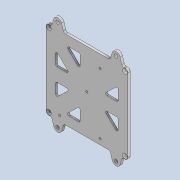
# Autodesk Inventor part: sacatola coperchio principale
Saved by Autodesk Inventor 2022 (Build 260153000, 153)
## iProperties
Created: 2025-07-12
Part Number: sacatola coperchio principale
Material: Generic
Document SubType Name: Modeling
Designer: 1234
Density: 1 g/cm^3
Appearance: Default
Author: 1234
Autodesk Inventor part; units mm, degrees
ref_plane "YZ Plane" through (0, 0, 0) normal (1, 0, 0) x (0, 1, 0)
ref_plane "XZ Plane" through (0, 0, 0) normal (0, 1, 0) x (-1, 0, 0)
ref_plane "XY Plane" through (0, 0, 0) normal (0, 0, 1) x (1, 0, 0)
sketch "Sketch1" plane through (0, 0, 0) normal (0, 0, 1) x (1, 0, 0)
  arc A0 (116, 108) -> (112, 112) centre (112, 108) ccw
  circle A1 centre (112, 108) radius 4 construction
  arc A2 (112, -4) -> (116, 0) centre (112, 0) ccw
  circle A3 centre (112, 0) radius 4 construction
  arc A4 (-4, 0) -> (0, -4) centre (0, 0) ccw
  circle A5 centre (0, 0) radius 4 construction
  arc A6 (0, 112) -> (-4, 108) centre (0, 108) ccw
  circle A7 centre (0, 108) radius 4 construction
  line L0 (0, 108) -> (112, 108) construction
  line L1 (112, 108) -> (112, 0) construction
  line L2 (112, 0) -> (0, 0) construction
  line L3 (0, 0) -> (0, 108) construction
  circle A8 centre (112, 0) radius 1.6
  circle A9 centre (0, 0) radius 1.6
  circle A10 centre (0, 108) radius 1.6
  circle A11 centre (112, 108) radius 1.6
  line L4 (116, 108) -> (116, 0)
  line L5 (112, 112) -> (0, 112)
  line L6 (-4, 108) -> (-4, 0)
  line L7 (0, -4) -> (112, -4)
  line L8 (6, -2) -> (106, -2)
  line L9 (106, -2) -> (6, -2)
  line L10 (-2, 6) -> (-2, 102)
  line L11 (-2, 6) -> (-2, 102)
  line L12 (106, 110) -> (6, 110)
  line L13 (6, 110) -> (106, 110)
  line L14 (114, 6) -> (114, 102)
  line L15 (114, 102) -> (114, 6)
  arc A12 (6, 110) -> (4, 108) centre (6, 108) ccw
  arc A13 (6, 110) -> (4, 108) centre (6, 108) ccw
  arc A14 (0, 104) -> (-2, 102) centre (0, 102) ccw
  arc A15 (0, 104) -> (4, 108) centre (0, 108) ccw
  arc A16 (0, 104) -> (4, 108) centre (0, 108) ccw
  arc A17 (0, 104) -> (-2, 102) centre (0, 102) ccw
  arc A18 (114, 102) -> (112, 104) centre (112, 102) ccw
  arc A19 (114, 102) -> (112, 104) centre (112, 102) ccw
  arc A20 (108, 108) -> (112, 104) centre (112, 108) ccw
  arc A21 (108, 108) -> (112, 104) centre (112, 108) ccw
  arc A22 (108, 108) -> (106, 110) centre (106, 108) ccw
  arc A23 (108, 108) -> (106, 110) centre (106, 108) ccw
  arc A24 (112, 4) -> (114, 6) centre (112, 6) ccw
  arc A25 (112, 4) -> (114, 6) centre (112, 6) ccw
  arc A26 (112, 4) -> (108, 0) centre (112, 0) ccw
  arc A27 (112, 4) -> (108, 0) centre (112, 0) ccw
  arc A28 (106, -2) -> (108, 0) centre (106, 0) ccw
  arc A29 (106, -2) -> (108, 0) centre (106, 0) ccw
  arc A30 (4, 0) -> (6, -2) centre (6, 0) ccw
  arc A31 (4, 0) -> (6, -2) centre (6, 0) ccw
  arc A32 (-2, 6) -> (0, 4) centre (0, 6) ccw
  arc A33 (-2, 6) -> (0, 4) centre (0, 6) ccw
  arc A34 (4, 0) -> (0, 4) centre (0, 0) ccw
  arc A35 (4, 0) -> (0, 4) centre (0, 0) ccw
  arc A36 (-0.5, 6) -> (0, 5.5) centre (0, 6) ccw
  line L16 (-0.5, 6) -> (-0.5, 102)
  arc A37 (0, 102.5) -> (-0.5, 102) centre (0, 102) ccw
  arc A38 (0, 102.5) -> (5.5, 108) centre (0, 108) ccw
  arc A39 (6, 108.5) -> (5.5, 108) centre (6, 108) ccw
  line L17 (6, 108.5) -> (106, 108.5)
  arc A40 (106.5, 108) -> (106, 108.5) centre (106, 108) ccw
  arc A41 (106.5, 108) -> (112, 102.5) centre (112, 108) ccw
  arc A42 (112.5, 102) -> (112, 102.5) centre (112, 102) ccw
  line L18 (112.5, 102) -> (112.5, 6)
  arc A43 (112, 5.5) -> (112.5, 6) centre (112, 6) ccw
  arc A44 (112, 5.5) -> (106.5, 0) centre (112, 0) ccw
  arc A45 (106, -0.5) -> (106.5, 0) centre (106, 0) ccw
  line L19 (106, -0.5) -> (6, -0.5)
  arc A46 (5.5, 0) -> (6, -0.5) centre (6, 0) ccw
  arc A47 (5.5, 0) -> (0, 5.5) centre (0, 0) ccw
  arc A48 (-1, 6) -> (0, 5) centre (0, 6) ccw
  line L20 (-1, 6) -> (-1, 102)
  arc A49 (0, 103) -> (-1, 102) centre (0, 102) ccw
  arc A50 (0, 103) -> (5, 108) centre (0, 108) ccw
  arc A51 (6, 109) -> (5, 108) centre (6, 108) ccw
  line L21 (6, 109) -> (106, 109)
  arc A52 (107, 108) -> (106, 109) centre (106, 108) ccw
  arc A53 (107, 108) -> (112, 103) centre (112, 108) ccw
  arc A54 (113, 102) -> (112, 103) centre (112, 102) ccw
  line L22 (113, 102) -> (113, 6)
  arc A55 (112, 5) -> (113, 6) centre (112, 6) ccw
  arc A56 (112, 5) -> (107, 0) centre (112, 0) ccw
  arc A57 (106, -1) -> (107, 0) centre (106, 0) ccw
  line L23 (106, -1) -> (6, -1)
  arc A58 (5, 0) -> (6, -1) centre (6, 0) ccw
  arc A59 (5, 0) -> (0, 5) centre (0, 0) ccw
  arc A60 (-2.5, 6) -> (0, 3.5) centre (0, 6) ccw
  line L24 (-2.5, 6) -> (-2.5, 102)
  arc A61 (0, 104.5) -> (-2.5, 102) centre (0, 102) ccw
  arc A62 (0, 104.5) -> (3.5, 108) centre (0, 108) ccw
  arc A63 (6, 110.5) -> (3.5, 108) centre (6, 108) ccw
  line L25 (6, 110.5) -> (106, 110.5)
  arc A64 (108.5, 108) -> (106, 110.5) centre (106, 108) ccw
  arc A65 (108.5, 108) -> (112, 104.5) centre (112, 108) ccw
  arc A66 (114.5, 102) -> (112, 104.5) centre (112, 102) ccw
  line L26 (114.5, 102) -> (114.5, 6)
  arc A67 (112, 3.5) -> (114.5, 6) centre (112, 6) ccw
  arc A68 (112, 3.5) -> (108.5, 0) centre (112, 0) ccw
  arc A69 (106, -2.5) -> (108.5, 0) centre (106, 0) ccw
  line L27 (106, -2.5) -> (6, -2.5)
  arc A70 (3.5, 0) -> (6, -2.5) centre (6, 0) ccw
  arc A71 (3.5, 0) -> (0, 3.5) centre (0, 0) ccw
  line L28 (111.5, 6.4807) -> (111.5, 101.5193)
  arc A72 (105.5193, 107.5) -> (111.5, 101.5193) centre (112, 108) ccw
  line L29 (105.5193, 107.5) -> (6.4807, 107.5)
  arc A73 (0.5, 101.5193) -> (6.4807, 107.5) centre (0, 108) ccw
  line L30 (0.5, 101.5193) -> (0.5, 6.4807)
  arc A74 (6.4807, 0.5) -> (0.5, 6.4807) centre (0, 0) ccw
  line L31 (6.4807, 0.5) -> (105.5193, 0.5)
  arc A75 (111.5, 6.4807) -> (105.5193, 0.5) centre (112, 0) ccw
  line L32 (111.5, 6.4807) -> (111.5, 101.5193)
  arc A76 (105.5193, 107.5) -> (111.5, 101.5193) centre (112, 108) ccw
  line L33 (105.5193, 107.5) -> (6.4807, 107.5)
  arc A77 (0.5, 101.5193) -> (6.4807, 107.5) centre (0, 108) ccw
  line L34 (0.5, 101.5193) -> (0.5, 6.4807)
  arc A78 (6.4807, 0.5) -> (0.5, 6.4807) centre (0, 0) ccw
  line L35 (6.4807, 0.5) -> (105.5193, 0.5)
  arc A79 (111.5, 6.4807) -> (105.5193, 0.5) centre (112, 0) ccw
  line L36 (-0.5, 8) -> (1.5, 8)
  line L37 (1.5, 8) -> (1.5, 13)
  line L38 (1.5, 13) -> (-0.5, 13)
  line L39 (7, -0.5) -> (7, 1.5)
  line L40 (7, 1.5) -> (12, 1.5)
  line L41 (12, 1.5) -> (12, -0.5)
  line L42 (-4, 54) -> (-11, 54) construction
  circle A80 centre (-11, 54) radius 1.7
  arc A81 (-11, 58) -> (-11, 50) centre (-11, 54) ccw
  line L43 (-11, 50) -> (-4, 50)
  line L44 (-11, 58) -> (-4, 58)
  line L45 (7, -4) -> (7, -13) construction
  arc A82 (7, -13) -> (19, -13) centre (13, -13) ccw
  line L46 (19, -13) -> (19, -4)
  circle A83 centre (13, -13) radius 2.6
  line L47 (22, -4) -> (18.7417, -14.7417)
  line L48 (7, -13) -> (7, -4)
  line L49 (4, -4) -> (7.2583, -14.7417)
  line L50 (-12.4444, 50.2699) -> (-4, 47)
  line L51 (-12.4444, 57.7301) -> (-4, 61)
  line L52 (7, 112) -> (7, 121) construction
  arc A84 (19, 121) -> (7, 121) centre (13, 121) ccw
  line L53 (19, 121) -> (19, 112)
  circle A85 centre (13, 121) radius 2.6
  line L54 (22, 112) -> (18.7417, 122.7417)
  line L55 (7, 121) -> (7, 112)
  line L56 (4, 112) -> (7.2583, 122.7417)
  line L57 (99, -0.5) -> (99, 1.5)
  line L58 (99, 1.5) -> (104, 1.5)
  line L59 (104, 1.5) -> (104, -0.5)
  line L60 (56, -4) -> (56, -8.0114) construction
  line L61 (116, 54) -> (127.5654, 54) construction
  line L62 (53.5, -0.5) -> (53.5, 1.5)
  line L63 (53.5, 1.5) -> (58.5, 1.5)
  line L64 (58.5, 1.5) -> (58.5, -0.5)
  line L65 (112.5, 8) -> (110.5, 8)
  line L66 (110.5, 8) -> (110.5, 13)
  line L67 (110.5, 13) -> (112.5, 13)
  line L68 (-0.5, 100) -> (1.5, 100)
  line L69 (1.5, 100) -> (1.5, 95)
  line L70 (1.5, 95) -> (-0.5, 95)
  line L71 (7, 108.5) -> (7, 106.5)
  line L72 (7, 106.5) -> (12, 106.5)
  line L73 (12, 106.5) -> (12, 108.5)
  line L74 (99, 108.5) -> (99, 106.5)
  line L75 (99, 106.5) -> (104, 106.5)
  line L76 (104, 106.5) -> (104, 108.5)
  line L77 (53.5, 108.5) -> (53.5, 106.5)
  line L78 (53.5, 106.5) -> (58.5, 106.5)
  line L79 (58.5, 106.5) -> (58.5, 108.5)
  line L80 (112.5, 100) -> (110.5, 100)
  line L81 (110.5, 100) -> (110.5, 95)
  line L82 (110.5, 95) -> (112.5, 95)
  line L83 (13, -13) -> (13, -6.0057) construction
  point P0 (0, 0)
  point P1 (0.5, 13)
  point P2 (0.5, 8)
  point P3 (12, 0.5)
  point P4 (7, 0.5)
  point P5 (0.5, 13)
  point P6 (0.5, 8)
  point P7 (12, 0.5)
  point P8 (7, 0.5)
  point P9 (4, 112)
  point P10 (22, 104)
  point P11 (111.5, 100)
  point P12 (104, 107.5)
  point P13 (104, 100.5)
  point P14 (0.5, 95)
  point P15 (0.5, 95)
  point P16 (0.5, 100)
  point P17 (0.5, 100)
  point P18 (7, 107.5)
  point P19 (7, 107.5)
  point P20 (12, 107.5)
  point P21 (12, 107.5)
  point P22 (53.5, 107.5)
  point P23 (53.5, 107.5)
  point P24 (58.5, 107.5)
  point P25 (58.5, 107.5)
  point P26 (99, 107.5)
  point P27 (99, 107.5)
  point P28 (104, 107.5)
  point P29 (111.5, 100)
  point P30 (111.5, 95)
  point P31 (111.5, 95)
  point P32 (111.5, 13)
  point P33 (111.5, 13)
  point P34 (111.5, 8)
  point P35 (111.5, 8)
  point P36 (104, 0.5)
  point P37 (104, 0.5)
  point P38 (99, 0.5)
  point P39 (99, 0.5)
  point P40 (58.5, 0.5)
  point P41 (58.5, 0.5)
  point P42 (53.5, 0.5)
  point P43 (53.5, 0.5)
  point P44 (99, 130.5)
  point P45 (104, 130.5)
  point P46 (99, 120.5)
  point P47 (104, 120.5)
  dimension "d15" = 8
  dimension "d16" = 8
  dimension "d18" = 8
  dimension "d19" = 8
  dimension "d0" = 3.2
  dimension "d1" = 3.2
  dimension "d2" = 3.2
  dimension "d3" = 3.2
  dimension "d9" = 1.5
  dimension "d10" = 0.5
  dimension "d11" = 1.5
  dimension "d12" = 108
  dimension "d20" = 3.5
  dimension "d22" = 2.5
  dimension "d23" = 3.5
  dimension "d24" = 2.5
  dimension "d25" = 2.5
  dimension "d26" = 3.5
  dimension "d27" = 2.5
  dimension "d28" = 3.5
  dimension "d29" = 2.5
  dimension "d30" = 2.5
  dimension "d40" = 1
  dimension "d45" = 1
  dimension "d48" = 8
  dimension "d49" = 5
  dimension "d50" = 5
  dimension "d64" = 7
  dimension "d65" = 3.4
  dimension "d66" = 8
  dimension "d67" = 12
  dimension "d68" = 9
  dimension "d69" = 5.2
  dimension "d74" = 3
  dimension "d81" = 3
  dimension "d82" = 3
  dimension "d83" = 3
  dimension "d95" = 2
  dimension "d96" = 2
  dimension "d100" = 2
  dimension "d101" = 5
  dimension "d102" = 8
  dimension "d106" = 4.0114
  dimension "d107" = 11.5654
  dimension "d108" = 2
  dimension "d109" = 5
  dimension "d110" = 2.5
  dimension "d111" = 2
  dimension "d112" = 5
  dimension "d113" = 8
  dimension "d145" = 112
  dimension "d154" = 13
  constraints: 168 end point, 158 point on circle, 82 centre point, 30 symmetric about line, 28 coincident, 27 point on line, 27 tangent, 13 perpendicular, 12 vertical, 11 horizontal, 3 equal length, 3 midpoint, 2 horizontal alignment, 2 vertical alignment, 1 concentric, 69 other
  measures "d0" diameter of A8
  measures "d1" diameter of A11
  measures "d2" diameter of A10
  measures "d3" diameter of A9
  measures "d9" radial gap between concentric circles of A34 A47
  measures "d10" radial gap between concentric circles of A47 A59
  measures "d11" radial gap between concentric circles of A59 A71
  measures "d12" distance of point (0, 0) L3.end
  measures "d20" radius of A68
  measures "d22" radius of A66
  measures "d23" radius of A65
  measures "d24" radius of A64
  measures "d25" radius of A63
  measures "d26" radius of A62
  measures "d27" radius of A61
  measures "d28" radius of A71
  measures "d29" radius of A60
  measures "d30" radius of A70
  measures "d40" distance between parallel lines of L18 L28
  measures "d45" distance between parallel lines of L18 L32
  measures "d48" distance from line of point (0, 0) L36
  measures "d49" distance of L36.end L37.end
  measures "d50" distance of L39.end L40.end
  measures "d64" distance of L42.start L42.end
  measures "d65" diameter of A80
  measures "d66" diameter of A81
  measures "d67" diameter of A82
  measures "d68" distance from line of A82.centre L7
  measures "d69" diameter of A83
  measures "d74" distance of L47.start L46.end
  measures "d81" distance from line of L45 L49.start
  measures "d82" distance of L50.end L43.end
  measures "d83" distance from line of L44 L51.end
  measures "d95" distance between parallel lines of L16 L37
  measures "d96" distance between parallel lines of L19 L40
  measures "d100" distance of L57.start L57.end
  measures "d101" distance of L57.end L58.end
  measures "d102" distance from line of A8.centre L59
  measures "d106" distance of L60.start L60.end
  measures "d107" distance of L61.start L61.end
  measures "d108" distance of L62.start L62.end
  measures "d109" distance of L62.end L63.end
  measures "d110" distance between parallel lines of L60 L62
  measures "d111" distance of L65.start L65.end
  measures "d112" distance of L65.end L66.end
  measures "d113" distance from line of L2.start L65
  measures "d145" distance of A16.centre A65.centre
  measures "d154" horizontal distance of point (0, 0) L83.end
extrude "Extrusion1" add sketch "Sketch1" along normal blind 4 contours L4 A2 L7 A4 L6 A6 L5 A0 | A30 A34 A32 L10 A14 A15 A12 L12 A22 A20 A18 L14 A24 A26 A28 L8 | L16 L36 L30 A74 L31 L39 L19 A46 A47 A36 | L16 L38 L30 L36 | L16 L70 L30 L38 | L36 L37 L38 L30 L70 L69 L68 A73 L29 L71 L72 L73 L77 L78 L79 L74 L75 L76 A72 L28 L80 L81 L82 L67 L66 L65 A75 L31 L59 L58 L57 L64 L63 L62 L41 L40 L39 A74 | L30 L38 L37 L36 | L16 L68 L30 L70 | L39 L31 L41 L19 | L16 A37 A38 A39 L17 L71 L29 A73 L30 L68 | L30 L68 L69 L70 | L41 L31 L62 L19 | L39 L40 L41 L31 | L62 L31 L64 L19 | L64 L31 L57 L19 | L62 L63 L64 L31 | L57 L31 L59 L19 | L71 L17 L73 L29 | L29 L73 L72 L71 | L59 L31 A75 L28 L65 L18 A43 A44 A45 L19 | L57 L58 L59 L31 | L73 L17 L77 L29 | L77 L17 L79 L29 | L29 L79 L78 L77 | L79 L17 L74 L29 | L74 L17 L76 L29 | L29 L76 L75 L74 | L65 L66 L67 L28 | L28 L67 L18 L65 | L76 L17 A40 A41 A42 L18 L80 L28 A72 L29 | L28 L82 L18 L67 | L82 L81 L80 L28 | L28 L80 L18 L82 | L20 A49 A50 A51 L21 A52 A53 A54 L22 A55 A56 A57 L23 A58 A59 A48 | L24 A61 A62 A63 L25 A64 A65 A66 L26 A67 A68 A69 L27 A70 A71 A60
chamfer "Chamfer1" distance 2 angle 45 4 edges at (-1.6, 108, 4) (-1.6, 0, 4) (110.4, 0, 4) (110.4, 108, 4)
extrude "Extrusion2" cut sketch "Sketch1" along normal blind 0.8 contours A30 A34 A32 L10 A14 A15 A12 L12 A22 A20 A18 L14 A24 A26 A28 L8 | L24 A61 A62 A63 L25 A64 A65 A66 L26 A67 A68 A69 L27 A70 A71 A60
extrude "Extrusion3" cut sketch "Sketch1" along normal blind 1.5 contours L16 L36 L30 A74 L31 L39 L19 A46 A47 A36 | L16 L38 L30 L36 | L16 L70 L30 L38 | L36 L37 L38 L30 L70 L69 L68 A73 L29 L71 L72 L73 L77 L78 L79 L74 L75 L76 A72 L28 L80 L81 L82 L67 L66 L65 A75 L31 L59 L58 L57 L64 L63 L62 L41 L40 L39 A74 | L30 L38 L37 L36 | L16 L68 L30 L70 | L39 L31 L41 L19 | L16 A37 A38 A39 L17 L71 L29 A73 L30 L68 | L30 L68 L69 L70 | L41 L31 L62 L19 | L39 L40 L41 L31 | L62 L31 L64 L19 | L64 L31 L57 L19 | L62 L63 L64 L31 | L57 L31 L59 L19 | L71 L17 L73 L29 | L29 L73 L72 L71 | L59 L31 A75 L28 L65 L18 A43 A44 A45 L19 | L57 L58 L59 L31 | L73 L17 L77 L29 | L77 L17 L79 L29 | L29 L79 L78 L77 | L79 L17 L74 L29 | L74 L17 L76 L29 | L29 L76 L75 L74 | L65 L66 L67 L28 | L28 L67 L18 L65 | L28 L82 L18 L67 | L82 L81 L80 L28 | L28 L80 L18 L82
ref_plane "Work Plane1" through (0, 0, 0.4) normal (0, 0, -1) x (-1, 0, 0)
extrude "Extrusion5" add sketch "Sketch1" along normal up to surface (1.5 mm away) contours L16 L36 L30 A74 L31 L39 L19 A46 A47 A36 | L16 L38 L30 L36 | L16 L70 L30 L38 | L16 L68 L30 L70 | L39 L31 L41 L19 | L16 A37 A38 A39 L17 L71 L29 A73 L30 L68 | L41 L31 L62 L19 | L62 L31 L64 L19 | L64 L31 L57 L19 | L57 L31 L59 L19 | L71 L17 L73 L29 | L59 L31 A75 L28 L65 L18 A43 A44 A45 L19 | L73 L17 L77 L29 | L77 L17 L79 L29 | L79 L17 L74 L29 | L74 L17 L76 L29 | L28 L67 L18 L65 | L76 L17 A40 A41 A42 L18 L80 L28 A72 L29 | L28 L82 L18 L67 | L28 L80 L18 L82
extrude "Extrusion8" add sketch "Sketch1" along normal up to surface (4 mm away) contours L5 L53 A84 L54 | L5 L55 A84 L53 | L47 A82 L46 L7 | L5 L56 A84 L55 | L46 A82 L48 L7 | L48 A82 L49 L7
ref_plane "Work Plane2" through (56, 0, 4) normal (1, 0, 0) x (0, 0, -1)
ref_plane "Work Plane3" through (0, 54, 4) normal (0, 1, 0) x (1, 0, 0)
fillet "Fillet2" radius 3 4 edges at (22, 112, 2) (4, 112, 2) (4, -4, 2) (22, -4, 2)
mirror "Mirror1" about plane through (56, 0, 4) normal (1, 0, 0) of "Extrusion8", "Fillet2"
sketch "Sketch4" plane through (0, 0, 1.5) normal (0, 0, -1) x (-1, 0, 0)
  arc A0 (-124.1209, 113.4267) -> (-124.3538, 112.9658) centre (-110, 106) ccw
  line L0 (-110, 106) -> (-2, 2) construction
  line L1 (-110, 2) -> (-2, 106) construction
  circle A1 centre (-56, 54) radius 1.5
  line L2 (-56, 54) -> (-56, 106) construction
  line L3 (-56, 54) -> (-56, 2) construction
  line L4 (-56, 54) -> (-2, 54) construction
  line L5 (-56, 54) -> (-110, 54) construction
  line L6 (-110.6936, 105.2797) -> (-2.6936, 1.2797)
  line L7 (-109.3064, 106.7203) -> (-1.3064, 2.7203)
  line L8 (-57, 17.0694) -> (-57, 106)
  line L9 (-55, 17.0694) -> (-55, 106)
  line L10 (-110.6936, 2.7203) -> (-2.6936, 106.7203)
  line L11 (-109.3064, 1.2797) -> (-1.3064, 105.2797)
  line L12 (-55, 17.0694) -> (-55, 2)
  line L13 (-57, 17.0694) -> (-57, 2)
  line L14 (-110.6936, 2.7203) -> (-109.3064, 1.2797)
  line L15 (-110.6936, 105.2797) -> (-109.3064, 106.7203)
  line L16 (-57, 106) -> (-55, 106)
  line L17 (-2.6936, 106.7203) -> (-1.3064, 105.2797)
  line L18 (-2.8786, 55) -> (-2, 55)
  line L19 (-2.4874, 53) -> (-2, 53)
  line L20 (-2.4874, 53) -> (-110, 53)
  line L21 (-2.5959, 55) -> (-110, 55)
  line L22 (-110, 55) -> (-110, 53)
  line L23 (-2, 53) -> (-2, 55)
  line L24 (-2.6936, 1.2797) -> (-1.3064, 2.7203)
  line L25 (-57, 2) -> (-55, 2)
  line L26 (-2, 2) -> (-2, 106) construction
  line L27 (-110, 106) -> (-110, 2) construction
  line L28 (-2, 106) -> (-110, 106) construction
  line L29 (-110, 2) -> (-2, 2) construction
  circle A2 centre (-112, 108) radius 1.6 projected
  line L30 (-112, 108) -> (-112, 84.3574) construction
  line L31 (-112, 108) -> (-118.8149, 108) construction
  line L32 (0, 0) -> (0, 31.7596) construction
  line L33 (0, 0) -> (-4.0584, 0) construction
  circle A3 centre (-112, 108) radius 6.5
  line L34 (-108.7987, 101.9536) -> (-106.5092, 104.3312)
  circle A4 centre (0, 108) radius 1.6 projected
  circle A5 centre (0, 108) radius 6.5
  line L35 (-3.4368, 102.1982) -> (-5.1252, 103.9515)
  circle A6 centre (0, 0) radius 1.6 projected
  circle A7 centre (0, 0) radius 6.5
  line L36 (-5.2223, 3.9477) -> (-3.1921, 6.056)
  circle A8 centre (-112, 0) radius 1.6 projected
  circle A9 centre (-112, 0) radius 6.5
  line L37 (-108.8312, 6.0802) -> (-106.6256, 3.7897)
  point P0 (-58.4801, 53)
  point P1 (-108.0486, 5.2674)
  point P2 (-106.6613, 3.8268)
  point P3 (-57, 51.6488)
  point P4 (-59.5, 2)
  point P5 (-57.5, 2)
  point P6 (-55, 51.6488)
  point P7 (-5.6797, 3.1867)
  point P8 (-3.9514, 5.2674)
  point P9 (-53.5199, 53)
  point P10 (-2, 37.5)
  point P11 (-2, 39.5)
  point P12 (-53.5199, 55)
  point P13 (-3.9514, 102.7326)
  point P14 (-5.6797, 73.8133)
  point P15 (-55, 56.3512)
  point P16 (-57, 56.3512)
  point P17 (-106.6613, 104.1732)
  point P18 (-108.0486, 102.7326)
  point P19 (-58.4801, 55)
  point P20 (-57, 54.4253)
  point P21 (-57.4417, 54)
  point P22 (-57, 53.5747)
  point P23 (-5.2888, 3.7787)
  point P24 (-3.8895, 5.2078)
  point P25 (-4.6821, 103.4913)
  point P26 (-5.2888, 104.2213)
  point P27 (-106.7112, 104.2213)
  point P28 (-108.1105, 102.7922)
  point P29 (-56, 52.6117)
  point P30 (-55, 55)
  point P31 (-55, 53)
  point P32 (-56, 55.3883)
  point P33 (-57, 53)
  point P34 (-57, 55)
  point P35 (-56.4032, 55)
  point P36 (-55.5968, 55)
  point P37 (-56.4032, 53)
  point P38 (-55.5968, 53)
  point P39 (-55, 53.5747)
  point P40 (-55, 54.4253)
  point P41 (-54.5583, 54)
  point P42 (-107.3179, 103.4913)
  point P43 (-108.1105, 5.2078)
  point P44 (-106.7112, 3.7787)
  dimension "d115" = 3
  dimension "d116" = 1
  dimension "d117" = 1
  dimension "d118" = 1
  dimension "d119" = 1
  dimension "d120" = 1
  dimension "d121" = 1
  dimension "d122" = 1
  dimension "d123" = 1
  dimension "d124" = 1
  dimension "d125" = 1
  dimension "d126" = 1
  dimension "d127" = 1
  dimension "d128" = 2
  dimension "d129" = 2
  dimension "d130" = 2
  dimension "d131" = 2
  dimension "d132" = 13
  dimension "d133" = 13
  dimension "d134" = 13
  dimension "d135" = 13
  constraints: 76 end point, 12 midpoint, 12 parallel, 9 perpendicular, 8 vertical, 6 centre point, 6 horizontal, 4 coincident, 4 collinear, 4 tangent, 2 point on circle
  measures "d115" diameter of A1
  measures "d116" distance between parallel lines of L0 L6
  measures "d117" distance between parallel lines of L0 L7
  measures "d118" distance between parallel lines of L2 L8
  measures "d119" distance between parallel lines of L2 L9
  measures "d120" distance between parallel lines of L1 L10
  measures "d121" distance between parallel lines of L1 L11
  measures "d122" distance between parallel lines of L3 L12
  measures "d123" distance between parallel lines of L3 L13
  measures "d124" distance between parallel lines of L4 L18
  measures "d125" distance between parallel lines of L4 L19
  measures "d126" distance between parallel lines of L5 L20
  measures "d127" distance between parallel lines of L5 L21
  measures "d128" distance between parallel lines of L30 L27
  measures "d129" distance between parallel lines of L31 L28
  measures "d130" distance between parallel lines of L33 L29
  measures "d131" distance between parallel lines of L26 L32
  measures "d132" diameter of A3
  measures "d133" diameter of A5
  measures "d134" diameter of A7
  measures "d135" diameter of A9
extrude "Extrusion9" cut sketch "Sketch4" against normal blind 1 contours A1 L7 L11 | A1 L11 L21 L18 L23 L19 L20 L7 | L11 L7 L9 L21 A1 | A1 L21 L11 | L7 L20 A1 | A1 L20 L9 L11 L7 | L21 L9 A1 | A1 L9 L10 A5 L35 L11 L21 | L11 L9 L7 | L20 L7 L36 A7 L6 L9 A1 | A1 L9 L20 | L9 L21 L7 L10 A1 | A1 L10 L9 | L9 L7 L21 | L9 L11 L20 L6 L8 L10 L21 L7 | L9 L20 L11 | L9 L6 A1 | A1 L6 L11 L20 L9 | L7 A7 L36 | L10 L7 A1 | A1 L7 L8 L16 L9 L10 | L21 L10 L7 | L11 L6 L20 | L6 L9 L12 L25 L13 L8 L11 A1 | A1 L11 L6 | L7 L10 L21 L8 A1 | A1 L8 L7 | L10 L8 L21 | L11 A1 L8 L20 L6 | L20 L8 L6 | L11 L8 A1 | L8 L21 A1 | A1 L21 L6 L34 L7 L8 | L10 L6 A1 L21 L8 | L8 L6 L10 | L8 L20 A1 L10 L6 | L8 A1 L20 | L8 L11 L37 L10 L20 A1 | A1 L6 L21 | L34 A3 L7 | L10 A1 L6 | L20 L10 A1 | L11 A9 L37 | A1 L10 L20 L22 L21 L6 | A9 L10 L37 | A2
extrude "Extrusion10" cut sketch "Sketch4" against normal through all contours A1 L7 L11 | L11 L7 L9 L21 A1 | A1 L20 L9 L11 L7 | L21 L9 A1 | L11 L9 L7 | A1 L9 L20 | L9 L21 L7 L10 A1 | L9 L7 L21 | L9 L11 L20 L6 L8 L10 L21 L7 | L9 L20 L11 | A1 L6 L11 L20 L9 | L10 L7 A1 | L21 L10 L7 | L11 L6 L20 | A1 L11 L6 | L7 L10 L21 L8 A1 | L10 L8 L21 | L11 A1 L8 L20 L6 | L20 L8 L6 | L8 L21 A1 | L10 L6 A1 L21 L8 | L8 L6 L10 | L8 L20 A1 L10 L6 | L8 A1 L20 | L10 A1 L6
fillet "Fillet4" radius 0.5 8 edges at (57, 56.3512, 2) (55, 56.3512, 2) (53.5199, 55, 2) (53.5199, 53, 2) (58.4801, 53, 2) (58.4801, 55, 2) (57, 51.6488, 2) (55, 51.6488, 2)
sketch "Sketch5" plane through (0, 0, 1.5) normal (0, 0, -1) x (-1, 0, 0)
  line L0 (-54.5, 53.3403) -> (-54.5, 98.5) construction
  circle A0 centre (-56, 54) radius 1.5 projected
  circle A1 centre (0, 0) radius 1.6 projected
  line L1 (-56, 54) -> (0, 0) construction
  line L2 (-56, 54) -> (0, 54) construction
  line L3 (0, 0) -> (0, 54) construction
  line L4 (-13.3883, 26.802) -> (-27.6561, 40.5603)
  line L5 (-26.2679, 44) -> (-12, 44)
  line L6 (-10, 42) -> (-10, 28.2417)
  arc A2 (-26.2679, 44) -> (-27.6561, 40.5603) centre (-26.2679, 42) ccw
  arc A3 (-10, 42) -> (-12, 44) centre (-12, 42) ccw
  arc A4 (-13.3883, 26.802) -> (-10, 28.2417) centre (-12, 28.2417) ccw
  line L7 (-56, 54) -> (-56, 0) construction
  line L8 (0, 0) -> (-56, 0) construction
  line L9 (-56, 54) -> (0, 0) construction
  line L10 (-28.3439, 13.4397) -> (-42.6117, 27.198)
  line L11 (-46, 25.7583) -> (-46, 12)
  line L12 (-44, 10) -> (-29.7321, 10)
  arc A5 (-42.6117, 27.198) -> (-46, 25.7583) centre (-44, 25.7583) ccw
  arc A6 (-46, 12) -> (-44, 10) centre (-44, 12) ccw
  arc A7 (-29.7321, 10) -> (-28.3439, 13.4397) centre (-29.7321, 12) ccw
  point P0 (-53.4138, 37)
  point P1 (-1.5, 37)
  point P2 (-54.5, 65)
  dimension "d157" = 10
  dimension "d158" = 2
  dimension "d159" = 10
  dimension "d160" = 2
  constraints: 24 end point, 12 point on circle, 12 tangent, 6 centre point, 4 equal radius, 2 horizontal, 2 vertical, 1 collinear, 5 other
  measures "d157" distance between parallel lines of L1 L4
  measures "d158" radius of A2
  measures "d159" distance between parallel lines of L1 L10
  measures "d160" radius of A5
extrude "Extrusion11" cut sketch "Sketch5" against normal through all contours L4 A2 L5 A3 L6 A4 | A7 L12 A6 L11 A5 L10
mirror "Mirror2" about plane through (56, 0, 4) normal (1, 0, 0) of "Extrusion11"
mirror "Mirror3" about plane through (0, 54, 4) normal (0, 1, 0) of "Extrusion11", "Mirror2"
chamfer "Chamfer8" distance 0.5 angle 45 28 edges at (57.3043, 57.0667, 1.5) (82.279, 80.694, 1.5) (57, 81.7634, 1.5) (29.721, 80.694, 1.5) (54.6957, 57.0667, 1.5) (55, 81.7634, 1.5) (28.289, 79.2964, 1.5) (52.7435, 55.313, 1.5) (27.1399, 55, 1.5) (27.1399, 53, 1.5) (52.7435, 52.687, 1.5) (28.2581, 28.6738, 1.5) (29.721, 27.306, 1.5) (54.6957, 50.9333, 1.5) (55, 26.2366, 1.5) (82.279, 27.306, 1.5) (57.3043, 50.9333, 1.5) (57, 26.2366, 1.5) (59.2565, 52.687, 1.5) (83.7419, 28.6738, 1.5) (84.8601, 53, 1.5) (59.2565, 55.313, 1.5) (84.8601, 55, 1.5) (83.711, 79.2964, 1.5) (56, 2, 1.5) (56, 106, 1.5) (110, 54, 1.5) (2, 54, 1.5)
sketch "Sketch6" plane through (0, 0, 1.5) normal (0, 0, -1) x (-1, 0, 0)
  line L0 (-12.505, 0.5) -> (-109, 0.5) construction
  line L1 (-109, 0.5) -> (-109, 96.995) construction
  circle A0 centre (-112, 0) radius 1.6 projected
  circle A1 centre (-75.485, 93.515) radius 1.4
  line L2 (-12.505, 0.5) -> (-12.505, 96.995) construction
  line L3 (-12.505, 96.995) -> (-109, 96.995) construction
  circle A2 centre (-75.485, 93.515) radius 4
  circle A3 centre (-75.485, 3.98) radius 1.4
  circle A4 centre (-75.485, 3.98) radius 4
  circle A5 centre (-15.985, 3.967) radius 1.4
  circle A6 centre (-15.985, 3.967) radius 4
  line L4 (-105.5193, 0.5) -> (-6.4807, 0.5) projected
  line L5 (-6.4807, 0.5) -> (-105.5193, 0.5)
  point P0 (0, 0)
  point P1 (-15.5891, -0.0134)
  point P2 (-73.5128, 0.5)
  point P3 (-77.4572, 0.5)
  point P4 (-13.99, 0.5)
  point P5 (-17.98, 0.5)
  dimension "d177" = 8
  dimension "d155" = 96.495
  dimension "d156" = 96.495
  dimension "d165" = 3
  dimension "d166" = 62.98
  dimension "d167" = 3.48
  dimension "d168" = 2.8
  dimension "d169" = 8
  dimension "d170" = 2.8
  dimension "d171" = 3.48
  dimension "d174" = 2.8
  dimension "d175" = 3.467
  dimension "d176" = 3.48
  dimension "d184" = 8
  dimension "d206" = 59.5
  constraints: 10 end point, 5 centre point, 3 coincident, 3 horizontal, 2 vertical, 1 perpendicular, 4 other
  measures "d155" distance of L0.end L1.end
  measures "d156" distance of L0.start L0.end
  measures "d165" distance from line of A0.centre L1
  measures "d166" distance from line of L2 A1.centre
  measures "d167" distance from line of L3 A1.centre
  measures "d168" diameter of A1
  measures "d169" diameter of A2
  measures "d170" diameter of A3
  measures "d171" distance from line of L0 A3.centre
  measures "d174" diameter of A5
  measures "d175" distance from line of L0 A5.centre
  measures "d176" distance from line of L2 A5.centre
  measures "d184" diameter of A4
  measures "d206" distance of A3.centre A5.centre
ref_plane "Work Plane4" through (0, 0, -5) normal (0, 0, -1) x (-1, 0, 0)
extrude "Extrusion12" add sketch "Sketch6" along normal up to surface (6.5 mm away) contours A2 | A4 L4 | A6 L4 picked at (-75.5413, 1.1967) picked at (-15.9287, 1.1924)
sketch "Sketch7" plane through (0, 0, 1.5) normal (0, 0, -1) x (-1, 0, 0)
  line L0 (-66, 10) -> (-87.2232, 10)
  line L1 (-87.2232, 10) -> (-66, 30.4652)
  line L2 (-66, 30.4652) -> (-66, 10)
  line L3 (-68, 10) -> (-82.2679, 10) projected
  line L4 (-66, 25.7583) -> (-66, 12) projected
  line L5 (-83.6561, 13.4397) -> (-69.3883, 27.198) projected
  line L6 (-66, 77.5348) -> (-66, 98)
  line L7 (-66, 98) -> (-87.2232, 98)
  line L8 (-87.2232, 98) -> (-66, 77.5348)
  line L9 (-69.3883, 80.802) -> (-83.6561, 94.5603) projected
  line L10 (-66, 96) -> (-66, 82.2417) projected
  line L11 (-82.2679, 98) -> (-68, 98) projected
  arc A0 (-5.2888, 3.7787) -> (-5.5681, 3.3535) centre (0, 0) ccw projected
  circle A1 centre (0, 0) radius 6.5
  line L12 (-14.1608, 11.628) -> (-12.0799, 13.789)
  line L13 (-12.0799, 13.789) -> (-3.4689, 5.4969)
  line L14 (-5.5681, 3.3535) -> (-14.1608, 11.628)
  arc A2 (-13.99, 0.5) -> (-17.98, 0.5) centre (-15.985, 3.967) ccw projected
  line L15 (-54.5, 50.4731) -> (-5.5681, 3.3535) projected
  point P0 (-68.1333, 98)
  point P1 (-72.9797, 98)
  point P2 (-5.5681, 3.3535)
  point P3 (-9.3564, -0.1)
  point P4 (-15.6536, -0.1)
  constraints: 18 end point, 7 collinear, 3 perpendicular, 2 point on circle, 1 centre point, 1 coincident, 1 horizontal, 1 parallel, 1 tangent, 1 vertical
extrude "Extrusion13" add sketch "Sketch7" against normal up to surface (2.5 mm away) contours L0 L1 L2 | L8 L7 L6 | A0 L14 L12 L13 A1
extrude "Extrusion14" cut sketch "Sketch6" against normal through all contours A1 | A3 | A5
sketch "Sketch8" plane through (-4, 0, 4) normal (-1, 0, 0) x (0, 0, 1)
  line L0 (-4, 0.5) -> (-9, 0.5) projected
  line L1 (-4, 0.5) -> (-4, 0.6)
  line L2 (-4, 0.6) -> (-9, 1.5)
  line L3 (-2.5, 0.5) -> (-4, 0.5) projected
  line L4 (-4, 0.5) -> (-9, 0.5) projected
  line L5 (-9, 0.5) -> (-9, 8.8609) construction
  line L6 (-9, 5.367) -> (-9, 2.567) projected
  line L7 (-9, 1.5) -> (-9, 0.5)
  line L8 (-9, 0.5) -> (-4, 0.5)
  line L9 (-4, 108) -> (-4, 0) projected
  point P0 (-9, 0.5)
  dimension "d192" = 0.1
  dimension "d197" = 1
  constraints: 10 end point, 4 collinear, 1 vertical
  measures "d192" distance of L0.start L1.end
  measures "d197" distance from line of L0 L2.end
extrude "Extrusion15" cut sketch "Sketch8" against normal up to surface (111 mm away) from surface at -4.5
sketch "Sketch9" plane through (0, 0, 0) normal (0, 0, -1) x (-1, 0, 0)
  line L0 (4, 112) -> (-116, 112)
  line L1 (-116, 112) -> (-116, -4)
  line L2 (-116, -4) -> (4, -4)
  line L3 (4, -4) -> (4, 112)
  line L4 (-116, 0) -> (-116, 108) projected
  line L5 (-110.225, -4) -> (-112, -4) projected
  line L6 (4, 108) -> (4, 0) projected
  line L7 (-1.775, 112) -> (0, 112) projected
  line L8 (4, 128.7396) -> (-117.6206, 128.7396)
  line L9 (-117.6206, 128.7396) -> (-117.6206, -19.4937)
  line L10 (-117.6206, -19.4937) -> (4, -19.4937)
  line L11 (4, -19.4937) -> (4, 128.7396)
  point P0 (0, 0)
  point P1 (4, -4)
  constraints: 16 end point, 4 collinear, 4 parallel, 2 horizontal, 2 perpendicular
extrude "Extrusion16" cut sketch "Sketch9" against normal blind 0.5 contours L0 L1 L2 L11 L10 L9 L8
chamfer "Chamfer12" distance 0.5 angle 45 8 edges at (56, -4, 0) (114.8284, -2.8284, 0) (116, 54, 0) (114.8284, 110.8284, 0) (56, 112, 0) (-2.8284, 110.8284, 0) (-4, 54, 0) (-2.8284, -2.8284, 0)
equation "\"d1\" = d0"
equation "\"d2\" = d0"
equation "\"d3\" = d0"
body "Solid1"
